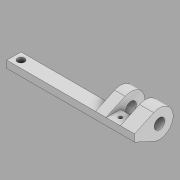
# Autodesk Inventor part: rocker
Saved by Autodesk Inventor 2020 (Build 240168000, 168)
## iProperties
Created: 2019-12-06
Part Number: rocker
Material: Generic
Document SubType Name: Modeling
Designer: alons
Density: 1 g/cm^3
Appearance: Default
Author: alons
Autodesk Inventor part; units mm, degrees
ref_plane "YZ Plane" through (0, 0, 0) normal (1, 0, 0) x (0, 1, 0)
ref_plane "XZ Plane" through (0, 0, 0) normal (0, 1, 0) x (-1, 0, 0)
sketch "Sketch1" plane through (0, 0, 0) normal (0, 1, 0) x (-1, 0, 0)
  point P0 (0, 0)
sketch "Sketch2" plane through (0, 0, 0) normal (1, 0, 0) x (0, 1, 0)
  point P0 (0, 0)
sketch "Sketch3" plane through (0, 0, 0) normal (1, 0, 0) x (0, 1, 0)
  line L0 (0, 0) -> (0.5, 0)
  line L1 (0.5, 0) -> (0.5, 1)
  line L2 (0.5, 1) -> (0, 1)
  line L3 (0, 1) -> (0, 0)
  dimension "d0" = 0.5
  dimension "d1" = 1
  constraints: 8 end point, 2 parallel, 1 horizontal, 1 perpendicular
  measures "d0" distance of L0.end L0.start
  measures "d1" distance of L0.start L2.end
extrude "Extrusion1" add sketch "Sketch3" along normal blind 9
sketch "Sketch4" plane through (9, 0, 0) normal (1, 0, 0) x (0, 0, -1)
  line L0 (0, 0) -> (0, 0.5) projected
  circle A0 centre (0.75, 0.25) radius 0.375
  line L1 (0, 0.5) -> (-1, 0.5) projected
  line L2 (-1, 0.5) -> (-1, 0) construction
  line L3 (-1, 0.25) -> (1.9779, 0.25) construction
  line L4 (0, 0) -> (0, 0.5) projected
  line L5 (0, 0.5) -> (-1, 0.5) projected
  line L6 (-1, 0.5) -> (-1, 0) projected
  line L7 (-1, 0) -> (0, 0) projected
  line L8 (-1, 0) -> (0, 0) projected
  line L9 (-1, 0.5) -> (0.3417, 1.1256)
  line L10 (-1, 0) -> (0.3417, -0.6256)
  arc A1 (0.3417, -0.6256) -> (0.3417, 1.1256) centre (0.75, 0.25) ccw
  point P0 (-0.5, 0)
  dimension "d9" = 0.75
  dimension "d12" = 1.25
  dimension "d13" = 0
  dimension "d14" = 25
  constraints: 6 end point, 2 centre point, 2 midpoint, 2 point on circle, 1 coincident, 1 equal length, 1 horizontal, 1 tangent
  measures "d9" diameter of A0
  measures "d12" horizontal distance of point (-0.5, 0) A1.centre
  measures "d13" vertical distance of A1.centre L3.start
  measures "d14" angle of L9 L1
extrude "Extrusion2" add sketch "Sketch4" against normal blind 1 contours L0 L1 L9 A1 L10 L7
ref_plane "Work Plane1" through (7, 0, 0) normal (-1, 0, 0) x (0, 0, 1)
sketch "Sketch5" plane through (7, 0, 0) normal (-1, 0, 0) x (0, 0, 1)
  line L0 (-0.3417, -0.6256) -> (1, 0) projected
  line L1 (0, 0) -> (1, 0) projected
  line L2 (0, 0.5) -> (0, 0) projected
  line L3 (1, 0.5) -> (0, 0.5) projected
  line L4 (1, 0.5) -> (-0.3417, 1.1256) projected
  arc A0 (-0.3417, 1.1256) -> (-0.3417, -0.6256) centre (-0.75, 0.25) ccw projected
  circle A1 centre (-0.75, 0.25) radius 0.375 projected
extrude "Extrusion3" add sketch "Sketch5" along normal blind 0.75
sketch "Sketch6" plane through (6.25, 0, 0) normal (-1, 0, 0) x (0, 0, 1)
  circle A0 centre (-0.75, 0.25) radius 0.375 projected
  point P0 (0, 0)
extrude "Extrusion4" add sketch "Sketch6" against normal blind 0.05
sketch "Sketch7" plane through (0, 0.5, 1) normal (0, 1, 0) x (1, 0, 0)
  line L0 (8, 2.6833) -> (9, 2.6833) projected
  line L1 (9, 2.6833) -> (9, 2.0295) projected
  line L2 (9, 2.0295) -> (8, 2.0295) projected
  line L3 (8, 2.0295) -> (8, 2.6833) projected
  line L4 (9, 0) -> (8, 0) projected
  line L5 (8, 0) -> (8, 1) projected
  line L6 (8, 1) -> (8, 1.4705) projected
  line L7 (8, 1.4705) -> (9, 1.4705) projected
  line L8 (9, 1.4705) -> (9, 0) projected
  line L9 (8, 0) -> (7, 0) projected
  line L10 (7, 1) -> (7, 0) projected
  line L11 (7, 1.4705) -> (7, 1) projected
  line L12 (6.3, 1.4705) -> (7, 1.4705) projected
  line L13 (6.3, 2.0295) -> (6.3, 1.4705) projected
  line L14 (7, 2.0295) -> (6.3, 2.0295) projected
  line L15 (7, 2.6833) -> (7, 2.0295) projected
  line L16 (6.25, 2.6833) -> (7, 2.6833) projected
  line L17 (6.25, 1) -> (6.25, 2.6833) projected
  line L18 (0, 1) -> (6.25, 1) projected
  line L19 (0, 0) -> (0, 1) projected
  line L20 (6.25, 0) -> (0, 0) projected
  line L21 (7, 0) -> (6.25, 0) projected
  line L22 (7, 1) -> (8, 1) projected
  line L23 (6.25, 0) -> (6.25, 1) projected
  circle A0 centre (7.5, 0.5) radius 0.5
  line L24 (7, 0) -> (8, 0) projected
  line L25 (7, 0) -> (7, 1.3417) projected
  line L26 (7, 1) -> (8, 1) projected
  line L27 (8, 0) -> (8, 1.3417) projected
  circle A1 centre (7.5, 0.5) radius 0.125
  line L28 (7, 0) -> (7.4116, 0.4116)
  line L29 (7.5884, 0.5884) -> (8, 1)
  line L30 (7, 1) -> (7.4116, 0.5884)
  line L31 (7.5884, 0.4116) -> (8, 0)
  dimension "d22" = 0.25
  constraints: 8 end point, 4 perpendicular, 4 point on circle, 4 tangent, 2 centre point, 1 point on line
  measures "d22" diameter of A1
extrude "Extrusion5" cut sketch "Sketch7" against normal through all contours A1
sketch "Sketch8" plane through (0, 0.5, 1) normal (0, 1, 0) x (1, 0, 0)
  line L0 (0, 1) -> (6.25, 1) projected
  line L1 (0, 0) -> (1, 0)
  line L2 (1, 0) -> (1, 1)
  line L3 (1, 1) -> (0, 1)
  line L4 (0, 1) -> (0, 0)
  line L5 (0, 1) -> (0, 0) projected
  circle A0 centre (0.5, 0.5) radius 0.25
  line L6 (0, 0) -> (0.3232, 0.3232)
  line L7 (0.6768, 0.6768) -> (1, 1)
  line L8 (0, 1) -> (0.3232, 0.6768)
  line L9 (0.6768, 0.3232) -> (1, 0)
  dimension "d25" = 1
  dimension "d26" = 0.5
  constraints: 16 end point, 4 point on circle, 2 parallel, 1 centre point, 1 horizontal, 1 perpendicular, 1 point on line
  measures "d25" distance of L2.end L0.start
  measures "d26" diameter of A0
extrude "Extrusion6" cut sketch "Sketch8" against normal through all contours A0
body "Solid1"
